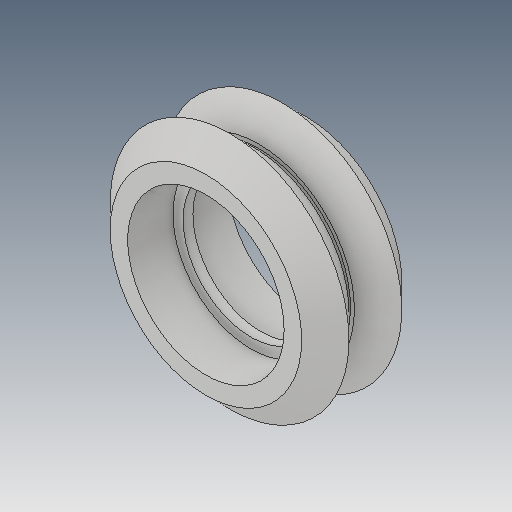
# Autodesk Inventor part: dELRIN
Saved by Autodesk Inventor 2017 (Build 210142000, 142)
## iProperties
Created: 2016-07-20
Part Number: dELRIN
Material: Generic
Document SubType Name: Modeling
Designer: User
Density: 1 g/cm^3
Appearance: Default
Mass: 1.83506 g
Surface Area: 18.2953 cm^2
Volume: 1.83506 cm^3
Author: User
Autodesk Inventor part; units mm, degrees
ref_plane "YZ Plane" through (0, 0, 0) normal (1, 0, 0) x (0, 1, 0)
ref_plane "XZ Plane" through (0, 0, 0) normal (0, 1, 0) x (-1, 0, 0)
ref_plane "XY Plane" through (0, 0, 0) normal (0, 0, 1) x (1, 0, 0)
sketch "Sketch1" plane through (0, 0, 0) normal (0, 0, 1) x (1, 0, 0)
  circle A0 centre (0, 0) radius 12.195
  dimension "d0" = 24.39
  constraints: 1 centre point, 1 coincident
  measures "d0" diameter of A0
extrude "Extrusion1" add sketch "Sketch1" along normal blind 10.23
sketch "Sketch2" plane through (0, 0, 0) normal (1, 0, 0) x (0, 1, 0)
  line L0 (-12.195, 0) -> (-12.195, 10.23) projected
  line L1 (9.375, 5.115) -> (9.375, 5.39)
  line L2 (9.375, 5.39) -> (9.375, 4.84)
  line L3 (9.375, 4.84) -> (9.375, 5.39)
  line L4 (12.195, 7.81) -> (9.775, 5.39)
  line L5 (12.195, 7.81) -> (15.6174, 7.81) construction
  line L6 (12.195, 7.81) -> (9.775, 10.23)
  line L7 (9.775, 4.84) -> (12.195, 2.42)
  line L8 (12.195, 2.42) -> (9.775, 0)
  line L9 (9.775, 4.84) -> (9.375, 4.84)
  line L10 (9.375, 5.39) -> (9.775, 5.39)
  line L11 (12.195, 7.81) -> (9.775, 10.23)
  line L12 (9.775, 10.23) -> (13.6006, 10.23)
  line L13 (13.6006, 10.23) -> (13.6006, 0)
  line L14 (13.6006, 0) -> (9.775, 0)
  line L15 (-12.195, 0) -> (12.195, 0) projected
  line L16 (0, -2.046) -> (0, 12.276) projected
  point P0 (0, 0)
  dimension "d4" = 0.275
  dimension "d5" = 0.55
  dimension "d6" = 135
  constraints: 28 end point, 2 collinear, 2 horizontal, 1 equal length, 1 parallel, 1 perpendicular, 1 point on line
  measures "d4" distance of L1.start L1.end
  measures "d5" distance of L1.end L2.end
  measures "d6" angle of L4 L5
revolve "Revolution1" cut sketch "Sketch2" angle 360 about axis through (0, 0, -10) along (0, 0, 1)
sketch "Sketch3" plane through (0, 0, 0) normal (0, 0, -1) x (-1, 0, 0)
  circle A0 centre (0, 0) radius 9.775 projected
  circle A1 centre (0, 0) radius 6.945
  dimension "d8" = 13.89
  constraints: 1 centre point, 1 coincident
  measures "d8" diameter of A1
extrude "Extrusion2" cut sketch "Sketch3" against normal blind 30 contours A1
sketch "Sketch4" plane through (0, 0, 0) normal (0, 0, -1) x (-1, 0, 0)
  circle A0 centre (0, 0) radius 7.987
  dimension "d11" = 15.974
  constraints: 1 centre point, 1 coincident
  measures "d11" diameter of A0
extrude "Extrusion3" cut sketch "Sketch4" against normal blind 4.615
sketch "Sketch5" plane through (0, 0, 10.23) normal (0, 0, 1) x (1, 0, 0)
  circle A0 centre (0, 0) radius 7.987
  dimension "d14" = 15.974
  constraints: 1 centre point, 1 coincident
  measures "d14" diameter of A0
extrude "Extrusion4" cut sketch "Sketch5" against normal blind 4.615
body "Solid1"
